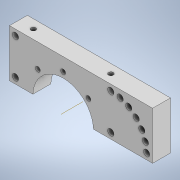
# Autodesk Inventor part: ShooterSeperableClampB
Saved by Autodesk Inventor 2020 (Build 240168000, 168)
## iProperties
Created: 2020-01-29
Part Number: ShooterSeperableClampB
Material: Generic
Document SubType Name: Modeling
Designer: srini
Density: 1 g/cm^3
Appearance: Default
Author: srini
Autodesk Inventor part; units mm, degrees
ref_plane "YZ Plane" through (0, 0, 0) normal (1, 0, 0) x (0, 1, 0)
ref_plane "XZ Plane" through (0, 0, 0) normal (0, 1, 0) x (-1, 0, 0)
ref_plane "XY Plane" through (0, 0, 0) normal (0, 0, 1) x (1, 0, 0)
sketch "Sketch1" plane through (0, 0, 0) normal (0, 0, 1) x (1, 0, 0)
  line L0 (76.2, -25.4) -> (-76.2, -25.4)
  line L1 (-76.2, -25.4) -> (-76.2, 25.4)
  line L2 (-76.2, 25.4) -> (76.2, 25.4)
  line L3 (76.2, 25.4) -> (76.2, -25.4)
  line L4 (76.2, -25.4) -> (-76.2, 25.4) construction
  line L5 (-76.2, -25.4) -> (76.2, 25.4) construction
  point P0 (0, 0)
  dimension "d0" = 50.8
  dimension "d1" = 152.4
  constraints: 12 end point, 2 midpoint, 2 parallel, 1 horizontal, 1 perpendicular
  measures "d0" distance of L0.end L1.end
  measures "d1" distance of L1.end L2.end
extrude "Extrusion1" add sketch "Sketch1" along normal blind 19.05
sketch "Sketch2" plane through (0, 0, 19.05) normal (0, 0, 1) x (1, 0, 0)
  line L0 (76.2, 25.4) -> (-76.2, 25.4) projected
  line L1 (-76.2, 25.4) -> (-76.2, -25.4) projected
  circle A0 centre (-19.05, -26.67) radius 32.258
  line L2 (-76.2, -25.4) -> (76.2, -25.4) projected
  point P0 (0, 0)
  dimension "d15" = 1.27
  dimension "d16" = 64.516
  dimension "d40" = 57.15
  constraints: 1 centre point
  measures "d15" distance from line of A0.centre L2
  measures "d16" diameter of A0
  measures "d40" distance from line of A0.centre L1
extrude "Extrusion2" cut sketch "Sketch2" against normal through all
sketch "Sketch3" plane through (-76.2, 25.4, 0) normal (0, 1, 0) x (1, 0, 0)
  circle A0 centre (15.875, -9.525) radius 2.5527
  line L0 (152.4, 0) -> (0, 0) projected
  circle A1 centre (98.425, -9.525) radius 2.5527
  line L1 (57.15, -22.86) -> (57.15, 3.81) projected
  dimension "d19" = 5.1054
  dimension "d20" = 9.525
  dimension "d24" = 82.55
  dimension "d41" = 41.275
  constraints: 2 centre point, 1 horizontal, 2 other
  measures "d19" diameter of A0
  measures "d20" distance from line of A0.centre L0
  measures "d24" distance of A0.centre A1.centre
  measures "d41" distance from line of A0.centre L1
extrude "Extrusion3" cut sketch "Sketch3" against normal through all
sketch "Sketch4" plane through (0, 0, 19.05) normal (0, 0, 1) x (1, 0, 0)
  circle A0 centre (-45.9908, 0.2708) radius 2.5797
  arc A1 (13.183, -25.4) -> (-51.283, -25.4) centre (-19.05, -26.67) ccw projected
  circle A2 centre (-19.05, 11.43) radius 2.5797
  circle A3 centre (7.8908, 0.2708) radius 2.5797
  line L0 (-19.05, -26.67) -> (-19.05, -17.7805)
  dimension "d31" = 5.1594
  dimension "d32" = 38.1
  dimension "d36" = 90
  dimension "d42" = 45
  constraints: 3 centre point, 2 end point, 1 vertical, 5 other
  measures "d31" diameter of A0
  measures "d32" distance of A0.centre L0.start
extrude "Extrusion4" cut sketch "Sketch4" against normal through all
sketch "Sketch5" plane through (0, 0, 19.05) normal (0, 0, 1) x (1, 0, 0)
  circle A0 centre (-69.85, -19.05) radius 3.3734
  arc A1 (13.183, -25.4) -> (-51.283, -25.4) centre (-19.05, -26.67) ccw projected
  line L0 (-76.2, -25.4) -> (-51.283, -25.4) projected
  line L1 (-76.2, 25.4) -> (-76.2, -25.4) projected
  circle A2 centre (-69.85, 19.05) radius 3.3734
  circle A3 centre (31.75, -19.05) radius 3.3734
  circle A4 centre (31.75, 19.05) radius 3.3734
  circle A5 centre (41.611, 17.7518) radius 3.3734
  circle A6 centre (50.8, 13.9456) radius 3.3734
  circle A7 centre (58.6908, 7.8908) radius 3.3734
  circle A8 centre (64.7456, 0) radius 3.3734
  circle A9 centre (68.5518, -9.189) radius 3.3734
  circle A10 centre (69.85, -19.05) radius 3.3734
  point P0 (0, 0)
  dimension "d43" = 6.7469
  dimension "d44" = 50.8
  dimension "d45" = 6.35
  dimension "d55" = 38.1
  dimension "d58" = 101.6
  dimension "d63" = 90
  constraints: 10 centre point, 1 horizontal, 1 vertical, 19 other
  measures "d43" diameter of A0
  measures "d44" horizontal distance of A0.centre A1.centre
  measures "d45" distance from line of A0.centre L0
  measures "d55" distance of A0.centre A2.centre
  measures "d58" distance of A0.centre A3.centre
extrude "Extrusion5" cut sketch "Sketch5" against normal through all
equation "\"d24\" = 2 * d41"
equation "\"d58\" = 2 * d44"
body "Solid1"
